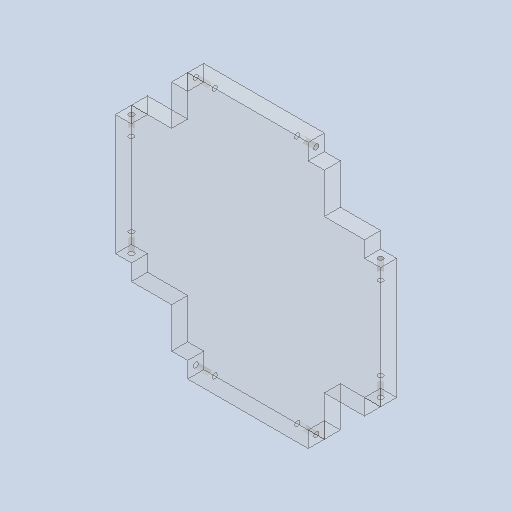
# Autodesk Inventor part: gearbox_cap
Saved by Autodesk Inventor 2023 (Build 270158000, 158)
## iProperties
Created: 2023-07-11
Part Number: gearbox_cap
Material: PMMA Plastic
Document SubType Name: Modeling
Designer: 310611102
Density: 1.188 g/cm^3
Appearance: Polycarbonate - Clear
Mass: 254.766 g
Surface Area: 506.225 cm^2
Volume: 214.449 cm^3
Author: 310611102
Autodesk Inventor part; units mm, degrees
ref_plane "YZ Plane" through (0, 0, 0) normal (1, 0, 0) x (0, 1, 0)
ref_plane "XZ Plane" through (0, 0, 0) normal (0, 1, 0) x (-1, 0, 0)
ref_plane "XY Plane" through (0, 0, 0) normal (0, 0, 1) x (1, 0, 0)
sketch "Sketch1" plane through (0, 0, 0) normal (0, 0, 1) x (1, 0, 0)
  line L0 (0, 82.5) -> (37.5, 82.5)
  line L1 (37.5, 82.5) -> (37.5, 72.5)
  line L2 (37.5, 72.5) -> (47.5, 72.5)
  line L3 (0, 101.1294) -> (0, 0)
  line L4 (0, 0) -> (69.4378, 0)
  line L5 (72.5, 47.5) -> (72.5, 37.5)
  line L6 (72.5, 37.5) -> (82.5, 37.5)
  line L7 (82.5, 37.5) -> (82.5, 0)
  line L8 (47.5, 72.5) -> (47.5, 47.5)
  line L9 (47.5, 47.5) -> (72.5, 47.5)
  line L10 (-82.5, 0) -> (-82.5, 37.5)
  line L11 (-82.5, 37.5) -> (-72.5, 37.5)
  line L12 (-72.5, 37.5) -> (-72.5, 47.5)
  line L13 (0, 0) -> (0, 69.4378)
  line L14 (-47.5, 72.5) -> (-37.5, 72.5)
  line L15 (-37.5, 72.5) -> (-37.5, 82.5)
  line L16 (-37.5, 82.5) -> (0, 82.5)
  line L17 (-72.5, 47.5) -> (-47.5, 47.5)
  line L18 (-47.5, 47.5) -> (-47.5, 72.5)
  line L19 (0, -82.5) -> (-37.5, -82.5)
  line L20 (-37.5, -82.5) -> (-37.5, -72.5)
  line L21 (-37.5, -72.5) -> (-47.5, -72.5)
  line L22 (0, 0) -> (-69.4378, 0)
  line L23 (-72.5, -47.5) -> (-72.5, -37.5)
  line L24 (-72.5, -37.5) -> (-82.5, -37.5)
  line L25 (-82.5, -37.5) -> (-82.5, 0)
  line L26 (-47.5, -72.5) -> (-47.5, -47.5)
  line L27 (-47.5, -47.5) -> (-72.5, -47.5)
  line L28 (82.5, 0) -> (82.5, -37.5)
  line L29 (82.5, -37.5) -> (72.5, -37.5)
  line L30 (72.5, -37.5) -> (72.5, -47.5)
  line L31 (0, 0) -> (0, -69.4378)
  line L32 (47.5, -72.5) -> (37.5, -72.5)
  line L33 (37.5, -72.5) -> (37.5, -82.5)
  line L34 (37.5, -82.5) -> (0, -82.5)
  line L35 (72.5, -47.5) -> (47.5, -47.5)
  line L36 (47.5, -47.5) -> (47.5, -72.5)
  point P0 (0, 50.5647)
  point P1 (-50.5647, 0)
  point P2 (0, -50.5647)
  point P3 (50.5647, 0)
  point P4 (82.5, 0)
  dimension "d0" = 75
  dimension "d1" = 165
  dimension "d2" = 10
  dimension "d3" = 10
  dimension "d4" = 165
  dimension "d5" = 75
  dimension "d25" = 10
  dimension "d26" = 10
  dimension "d29" = 360
  constraints: 74 end point, 4 perpendicular, 3 horizontal, 3 vertical, 2 coincident, 1 midpoint, 83 other
  measures "d0" diameter of L1 L3
  measures "d1" diameter of L0 L4
  measures "d2" distance of L0.end L1.end
  measures "d3" distance of L5.end L6.end
  measures "d4" diameter of L7 point (0, 50.565)
  measures "d5" diameter of L6 L4
  measures "d25" distance of L1.end L2.end
  measures "d26" distance of L5.start L5.end
extrude "Extrusion1" add sketch "Sketch1" along normal blind 10
sketch "Sketch2" plane through (37.5, 72.5, 0) normal (1, 0, 0) x (0, 0, -1)
  circle A0 centre (-5, 5) radius 2
  line L0 (0, 0) -> (0, 10) projected
  line L1 (0, 10) -> (-10, 10) projected
  point P0 (0, -72.5)
  dimension "d12" = 4
  dimension "d13" = 5
  dimension "d14" = 5
  constraints: 1 centre point
  measures "d12" diameter of A0
  measures "d13" distance from line of L0 A0.centre
  measures "d14" distance from line of L1 A0.centre
hole "Hole1" at (37.5, 77.5, 5) direction (-1, 0, 0) diameter 3.242 depth 11.8 tip angle 118 thread size "M4x0.7" class "6H" standard "ISO Metric profile"
mirror "Mirror1" about plane through (0, 0, 0) normal (1, 0, 0) of "Hole1"
pattern_circular "Circular Pattern1" count 4 over 360 about axis through (0, 0, -10) along (0, 0, 1) of "Hole1", "Mirror1"
body "Solid1"
